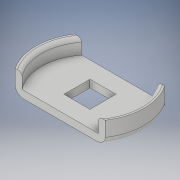
# Autodesk Inventor part: Battery_Holder
Saved by Autodesk Inventor 2019.4 (Build 234330000, 330)
## iProperties
Created: 2020-03-14
Part Number: Battery_Holder
Material: Generic
Document SubType Name: Modeling
Designer: Jorian Brusind
Density: 1 g/cm^3
Appearance: Default
Author: Jorian Brusind
Autodesk Inventor part; units mm, degrees
ref_plane "YZ Plane" through (0, 0, 0) normal (1, 0, 0) x (0, 1, 0)
ref_plane "XZ Plane" through (0, 0, 0) normal (0, 1, 0) x (-1, 0, 0)
ref_plane "XY Plane" through (0, 0, 0) normal (0, 0, 1) x (1, 0, 0)
sketch "Sketch1" plane through (0, 0, 0) normal (0, 1, 0) x (-1, 0, 0)
  circle A0 centre (0, 0) radius 13
  circle A1 centre (0, 0) radius 14.5
  dimension "d0" = 26
  dimension "d1" = 29
  constraints: 2 centre point, 2 coincident
  measures "d0" diameter of A0
  measures "d1" diameter of A1
extrude "Extrusion1" add sketch "Sketch1" along normal blind 4
sketch "Sketch2" plane through (0, 0, 0) normal (0, -1, 0) x (1, 0, 0)
  circle A0 centre (0, 0) radius 14.5
  dimension "d4" = 29
  constraints: 1 centre point, 1 coincident
  measures "d4" diameter of A0
extrude "Extrusion2" add sketch "Sketch2" along normal blind 2
sketch "Sketch3" plane through (0, 0, 0) normal (0, 1, 0) x (1, 0, 0)
  line L0 (-3.5, 3.5) -> (3.5, 3.5)
  line L1 (3.5, 3.5) -> (3.5, -3.5)
  line L2 (3.5, -3.5) -> (-3.5, -3.5)
  line L3 (-3.5, -3.5) -> (-3.5, 3.5)
  line L4 (-3.5, 3.5) -> (3.5, -3.5) construction
  line L5 (3.5, 3.5) -> (-3.5, -3.5) construction
  point P0 (0, 0)
  dimension "d7" = 7
  dimension "d8" = 7
  constraints: 12 end point, 2 midpoint, 2 parallel, 1 horizontal, 1 perpendicular
  measures "d7" distance of L1.end L2.end
  measures "d8" distance of L0.end L1.end
extrude "Extrusion3" cut sketch "Sketch3" against normal blind 3
fillet "Fillet1" radius 2 1 edges at (-14.5, -2, 0)
fillet "Fillet2" radius 1 1 edges at (13, 4, 0)
sketch "Sketch4" plane through (0, 0, 0) normal (0, 1, 0) x (1, 0, 0)
  line L0 (0, 0) -> (0, -8)
  line L1 (0, 0) -> (0, 8)
  line L2 (0, 8) -> (16, 8)
  line L3 (16, 8) -> (16, 16)
  line L4 (0, 8) -> (0, 12)
  line L5 (0, 8) -> (4, 8) construction
  line L6 (-16, 16) -> (16, 16)
  line L7 (16, 16) -> (16, 8)
  line L8 (16, 8) -> (-16, 8)
  line L9 (-16, 8) -> (-16, 16)
  line L10 (-16, 16) -> (16, 8) construction
  line L11 (16, 16) -> (-16, 8) construction
  line L12 (0, -8) -> (0, -12)
  line L13 (-16, -8) -> (16, -8)
  line L14 (16, -8) -> (16, -16)
  line L15 (16, -16) -> (-16, -16)
  line L16 (-16, -16) -> (-16, -8)
  line L17 (-16, -8) -> (16, -16) construction
  line L18 (16, -8) -> (-16, -16) construction
  dimension "d13" = 8
  dimension "d14" = 8
  dimension "d15" = 16
  dimension "d16" = 8
  dimension "d17" = 4
  dimension "d18" = 90
  dimension "d19" = 4
  dimension "d20" = 32
  dimension "d21" = 8
  constraints: 38 end point, 4 horizontal, 4 midpoint, 4 parallel, 4 perpendicular, 4 vertical
  measures "d13" distance of L0.start L0.end
  measures "d14" distance of L0.start L1.end
  measures "d15" distance of L1.end L2.end
  measures "d16" distance of L2.end L3.end
  measures "d17" distance of L1.end L4.end
  measures "d18" angle of L5 L4
  measures "d19" distance of L0.end L12.end
  measures "d20" distance of L14.end L15.end
  measures "d21" distance of L13.end L14.end
extrude "Extrusion4" cut sketch "Sketch4" along normal mid plane 20
body "Solid1"
